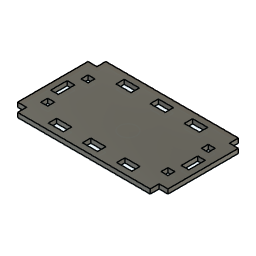
PiastraBaseScatolaGrande v3 (Autodesk Fusion 360 design; units mm, degrees)
Autodesk Fusion 360 part; units mm, degrees
sketch "Schizzo1" plane through (0, 0, 0) normal (0, 0, 1) x (1, 0, 0)
  line L0 (0, 0) -> (220, 0)
  line L1 (220, 0) -> (220, 129)
  line L2 (220, 129) -> (0, 129)
  line L3 (0, 129) -> (0, 0)
  line L4 (0, 129) -> (9, 129)
  line L5 (9, 129) -> (9, 0)
  line L6 (220, 129) -> (210, 129)
  line L7 (210, 129) -> (210, 0)
  line L8 (20, 129) -> (20, 0)
  line L9 (210, 64.5) -> (200, 64.5)
  line L10 (200, 129) -> (200, 0)
  line L11 (9, 64.5) -> (20, 64.5)
  line L12 (20, 64.5) -> (20, 76.5)
  line L13 (20, 64.5) -> (20, 52.5)
  line L14 (20, 76.5) -> (9, 76.5)
  line L15 (20, 52.5) -> (9, 52.5)
  line L16 (0, 129) -> (17, 129)
  line L17 (17, 129) -> (17, 99)
  line L18 (17, 99) -> (27, 99)
  line L19 (27, 99) -> (27, 89)
  line L20 (27, 89) -> (17, 89)
  line L21 (17, 89) -> (17, 99)
  line L22 (0, 129) -> (49, 129)
  line L23 (0, 129) -> (13, 129)
  line L24 (13, 129) -> (13, 116)
  line L25 (13, 116) -> (0, 116)
  line L26 (0, 116) -> (0, 129)
  line L27 (49, 129) -> (49, 120)
  line L28 (49, 120) -> (49, 108)
  line L29 (49, 108) -> (71, 108)
  line L30 (71, 108) -> (71, 120)
  line L31 (71, 120) -> (49, 120)
  line L32 (0, 129) -> (98, 129)
  line L33 (98, 129) -> (98, 120)
  line L34 (98, 120) -> (98, 108)
  line L35 (98, 108) -> (120, 108)
  line L36 (120, 108) -> (120, 120)
  line L37 (120, 120) -> (98, 120)
  line L38 (110, 0) -> (110, 129)
  line L39 (0, 64.5) -> (220, 64.5)
  line L40 (9, 76.5) -> (9, 52.5)
  line L41 (200, 76.5) -> (211, 76.5)
  line L42 (211, 76.5) -> (211, 52.5)
  line L43 (200, 64.5) -> (200, 76.5)
  line L44 (200, 64.5) -> (200, 52.5)
  line L45 (200, 52.5) -> (211, 52.5)
  line L46 (193, 99) -> (193, 89)
  line L47 (193, 89) -> (203, 89)
  line L48 (203, 89) -> (203, 99)
  line L49 (203, 99) -> (193, 99)
  line L50 (207, 116) -> (220, 116)
  line L51 (207, 129) -> (207, 116)
  line L52 (149, 120) -> (171, 120)
  line L53 (171, 108) -> (149, 108)
  line L54 (149, 108) -> (149, 120)
  line L55 (171, 120) -> (171, 108)
  line L56 (100, 120) -> (122, 120)
  line L57 (122, 120) -> (122, 108)
  line L58 (122, 108) -> (100, 108)
  line L59 (100, 108) -> (100, 120)
  line L60 (99, 120) -> (99, 108)
  line L61 (121, 108) -> (121, 120)
  circle A0 centre (110, 64.5) radius 12.5
  point P0 (49, 120)
  point P1 (98, 120)
  dimension "d1" = 220
  dimension "d2" = 129
  dimension "d3" = 9
  dimension "d4" = 10
  dimension "d6" = 12
  dimension "d7" = 12
  dimension "d8" = 17
  dimension "d9" = 30
  dimension "d10" = 10
  dimension "d11" = 10
  dimension "d12" = 49
  dimension "d13" = 13
  dimension "d14" = 13
  dimension "d15" = 9
  dimension "d16" = 12
  dimension "d17" = 22
  dimension "d18" = 98
  dimension "d19" = 9
  dimension "d20" = 12
  dimension "d21" = 22
  dimension "d28" = 25
  constraint horizontal L0
  constraint vertical L1
  constraint horizontal L2
  constraint vertical L3
  constraint coincident L0.start L3.end
  constraint perpendicular L3 L4
  constraint coincident L0 L5.end
  constraint perpendicular L0 L5
  constraint coincident L2 L6.end
  constraint coincident L0 L7.end
  constraint perpendicular L0 L7
  constraint coincident L2 L8.start
  constraint coincident L0 L8.end
  constraint perpendicular L0 L8
  constraint midpoint L7 L9.start
  constraint perpendicular L7 L9
  constraint coincident L2 L10.start
  constraint coincident L0 L10.end
  constraint perpendicular L0 L10
  constraint midpoint L5 L11.start
  constraint midpoint L8 L11.end
  constraint coincident L8 L12.end
  constraint perpendicular L11 L12
  constraint coincident L8 L13.end
  constraint coincident L5 L14.end
  constraint perpendicular L5 L14
  constraint coincident L5 L15.end
  constraint perpendicular L5 L15
  constraint coincident L2 L16.end
  constraint perpendicular L2 L17
  constraint perpendicular L8 L18
  constraint perpendicular L18 L19
  constraint perpendicular L8 L20
  constraint perpendicular L18 L21
  constraint coincident L2 L22.end
  constraint horizontal L23
  constraint vertical L24
  constraint horizontal L25
  constraint vertical L26
  constraint perpendicular L22 L27
  constraint perpendicular L22 L28
  constraint perpendicular L28 L29
  constraint perpendicular L29 L30
  constraint perpendicular L28 L31
  constraint coincident L2 L32.end
  constraint perpendicular L32 L33
  constraint perpendicular L32 L34
  constraint perpendicular L34 L35
  constraint perpendicular L32 L36
  constraint perpendicular L33 L37
  constraint midpoint L0 L38.start
  constraint midpoint L2 L38.end
  constraint midpoint L3 L39.start
  constraint midpoint L1 L39.end
  constraint coincident P0 L27.end
  constraint coincident P1 L33.end
  constraint symmetric L11.end L38 L9.end
  constraint symmetric L12.end L38 L41.start
  constraint symmetric L13.end L38 L44.end
  constraint symmetric L14.end L38 L41.end
  constraint symmetric L15.end L38 L42.end
  constraint symmetric L17.end L38 L48.end
  constraint symmetric L18.end L38 L46.start
  constraint symmetric L19.end L38 L46.end
  constraint symmetric L20.end L38 L47.end
  constraint symmetric L23.end L38 L51.start
  constraint symmetric L24.end L38 L50.start
  constraint symmetric L25.end L38 L50.end
  constraint symmetric P0 L38 L52.end
  constraint symmetric L28.end L38 L53.start
  constraint symmetric L29.end L38 L53.end
  constraint symmetric L30.end L38 L52.start
  constraint symmetric P1 L38 L56.end
  constraint symmetric L34.end L38 L57.end
  constraint symmetric L35.end L38 L58.end
  constraint symmetric L36.end L38 L56.start
  constraint coincident L37 L60.start
  constraint coincident L35 L60.end
  constraint perpendicular L35 L60
  constraint coincident L58 L61.start
  constraint coincident L56 L61.end
  constraint perpendicular L56 L61
  constraint midpoint L38 A0.centre
  measures "d1" distance of L0.start L0.end
  measures "d2" distance of L0.start L2.end
  measures "d3" distance of L2.end L4.end
  measures "d4" distance of L1.end L6.end
  measures "d6" distance of L11.end L12.end
  measures "d7" distance of L11.end L13.end
  measures "d8" distance of L2.end L16.end
  measures "d9" distance of L16.end L17.end
  measures "d10" distance of L17.end L18.end
  measures "d11" distance of L18.end L19.end
  measures "d12" distance of L2.end L22.end
  measures "d13" distance of L2.end L23.end
  measures "d14" distance of L2.end L25.end
  measures "d15" distance of L22.end P0
  measures "d16" distance of P0 L28.end
  measures "d17" distance of L28.end L29.end
  measures "d18" distance of L2.end L32.end
  measures "d19" distance of L32.end P1
  measures "d20" distance of P1 L34.end
  measures "d21" distance of L34.end L35.end
  measures "d28" diameter of A0
extrude "Estrusione1" add sketch "Schizzo1" along normal blind 6.5 contours L3 L5 L25 L39 L40 | L2 L5 L8 L14 L16 L17 L20 L21 L22 L24 L25 L32 | L2 L8 L12 L18 L19 L20 L22 L32 L33 L34 L35 L38 L39 L58 A0 | L38 L39 A0 | L38 L39 A0 | L2 L10 L35 L37 L38 L39 L43 L46 L47 L49 L56 L57 L58 A0 | L2 L8 L17 L18 L22 L32 | L1 L7 L39 L41 L42 L50 | L2 L7 L10 L41 L47 L48 L49 L50 L51 | L2 L33 L37 L38 L56 | L34 L35 L37 L60 | L56 L57 L58 L61 picked at (101.7091, 65.093) picked at (113.9836, 71.7954) makes body 1
mirror "Specchio1" about plane through (20, 64.5, 0) normal (0, -1, 0) of bodies 1 merged
extrude "Estrusione3" cut sketch "Schizzo1" along normal blind 2.5 contours L38 L39 A0 | L38 L39 A0 | L38 L39 A0 | L38 L39 A0 bodies 1
extrude "Estrusione4" add 1 faces at (50.5, 64.5, 0) along direction (0, 0, -1) blind 0.5 separate body on bodies 1 makes body 2
sketch "Schizzo2" plane through (0, 0, -0.5) normal (0, 0, -1) x (1, 0, 0)
  circle A0 centre (110, -64.5) radius 12.5
  line L0 (20, -52.5) -> (20, -76.5)
  line L1 (20, -76.5) -> (9, -76.5)
  line L2 (9, -76.5) -> (9, -52.5)
  line L3 (9, -52.5) -> (20, -52.5)
  line L4 (0, -13) -> (0, -116)
  line L5 (0, -116) -> (13, -116)
  line L6 (13, -116) -> (13, -129)
  line L7 (13, -129) -> (207, -129)
  line L8 (207, -129) -> (207, -116)
  line L9 (207, -116) -> (220, -116)
  line L10 (220, -116) -> (220, -13)
  line L11 (220, -13) -> (207, -13)
  line L12 (207, -13) -> (207, 0)
  line L13 (207, 0) -> (13, 0)
  line L14 (13, 0) -> (13, -13)
  line L15 (13, -13) -> (0, -13)
  line L16 (27, -40) -> (17, -40)
  line L17 (17, -40) -> (17, -30)
  line L18 (17, -30) -> (27, -30)
  line L19 (27, -30) -> (27, -40)
  line L20 (121, -21) -> (99, -21)
  line L21 (99, -21) -> (99, -9)
  line L22 (99, -9) -> (121, -9)
  line L23 (121, -9) -> (121, -21)
  line L24 (193, -30) -> (203, -30)
  line L25 (203, -30) -> (203, -40)
  line L26 (203, -40) -> (193, -40)
  line L27 (193, -40) -> (193, -30)
  line L28 (49, -9) -> (71, -9)
  line L29 (71, -9) -> (71, -21)
  line L30 (71, -21) -> (49, -21)
  line L31 (49, -21) -> (49, -9)
  line L32 (149, -9) -> (171, -9)
  line L33 (171, -9) -> (171, -21)
  line L34 (171, -21) -> (149, -21)
  line L35 (149, -21) -> (149, -9)
  line L36 (171, -120) -> (149, -120)
  line L37 (149, -120) -> (149, -108)
  line L38 (149, -108) -> (171, -108)
  line L39 (171, -108) -> (171, -120)
  line L40 (71, -120) -> (49, -120)
  line L41 (49, -120) -> (49, -108)
  line L42 (49, -108) -> (71, -108)
  line L43 (71, -108) -> (71, -120)
  line L44 (203, -99) -> (193, -99)
  line L45 (193, -99) -> (193, -89)
  line L46 (193, -89) -> (203, -89)
  line L47 (203, -89) -> (203, -99)
  line L48 (99, -108) -> (121, -108)
  line L49 (121, -108) -> (121, -120)
  line L50 (121, -120) -> (99, -120)
  line L51 (99, -120) -> (99, -108)
  line L52 (17, -89) -> (27, -89)
  line L53 (27, -89) -> (27, -99)
  line L54 (27, -99) -> (17, -99)
  line L55 (17, -99) -> (17, -89)
  line L56 (200, -76.5) -> (200, -52.5)
  line L57 (200, -52.5) -> (211, -52.5)
  line L58 (211, -52.5) -> (211, -76.5)
  line L59 (211, -76.5) -> (200, -76.5)
hidden bodies 2
named bodies: "BaseScatola", "StencilDimensioni"
